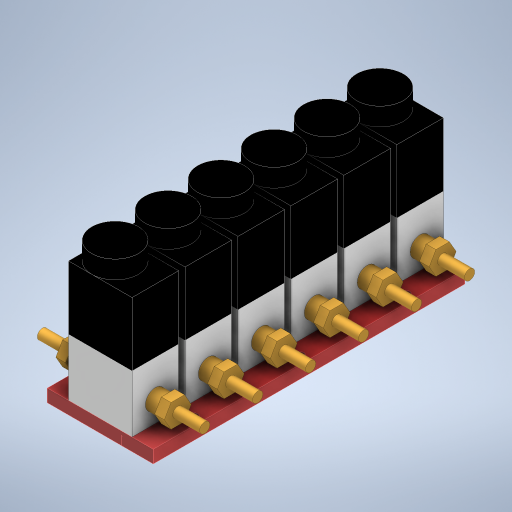
# Autodesk Inventor part: Montaje Valvulas
Saved by Autodesk Inventor 2024.2 (Build 282272000, 272)
## iProperties
Created: 2024-05-06
Part Number: Montaje Valvulas
Material: Generic
Document SubType Name: Modeling
Designer: jp.reyesf
Density: 1 g/cm^3
Appearance: Default
Author: jp.reyesf
Autodesk Inventor part; units mm, degrees
ref_plane "YZ Plane" through (0, 0, 0) normal (1, 0, 0) x (0, 1, 0)
sketch "Sketch1" plane through (0, 0, 0) normal (0, 1, 0) x (-1, 0, 0)
  line L0 (-15, 11) -> (15, 11)
  line L1 (15, 11) -> (15, -11)
  line L2 (15, -11) -> (-15, -11)
  line L3 (-15, -11) -> (-15, 11)
  line L4 (-15, 11) -> (15, -11) construction
  line L5 (15, 11) -> (-15, -11) construction
  line L6 (0, 0) -> (-10, 0)
  line L7 (-10, 7.5) -> (-10, -7.5) construction
  circle A0 centre (-10, 7.5) radius 1.7859
  circle A1 centre (-10, -7.5) radius 1.7859
  dimension "d0" = 22
  dimension "d1" = 30
  dimension "d2" = 15
  dimension "d3" = 5
  dimension "d4" = 3.5719
  constraints: 16 end point, 3 midpoint, 2 centre point, 2 coincident, 2 horizontal, 2 parallel, 1 equal radius, 1 perpendicular, 1 vertical
  measures "d0" distance of L0.end L1.end
  measures "d1" distance of L1.end L2.end
  measures "d2" distance of L7.start L7.end
  measures "d3" distance between parallel lines of L7 L3
  measures "d4" diameter of A0
extrude "Extrusion1" add sketch "Sketch1" along normal blind 27
sketch "Sketch2" plane through (0, 27, 0) normal (0, 1, 0) x (1, 0, 0)
  line L0 (15, 11) -> (-15, 11) projected
  line L1 (-15, 11) -> (-15, -11) projected
  line L2 (-15, -11) -> (15, -11) projected
  line L3 (15, -11) -> (15, 11) projected
  circle A0 centre (10, 7.5) radius 1.7859 projected
  circle A1 centre (10, -7.5) radius 1.7859 projected
  point P0 (0, 0)
extrude "Extrusion2" add sketch "Sketch2" along normal blind 30 separate body contours L3 L2 L1 L0 | A0 | A1
sketch "Sketch3" plane through (0, 57, 0) normal (0, 1, 0) x (1, 0, 0)
  circle A0 centre (-4, 0) radius 11
  line L0 (15, 11) -> (-15, 11) projected
  line L1 (-15, 11) -> (-15, -11) projected
  line L2 (-15, -11) -> (15, -11) projected
  point P0 (0, 0)
  constraints: 3 tangent, 1 centre point
extrude "Extrusion3" add sketch "Sketch3" along normal blind 8.5 contours A0 bodies 2
sketch "Sketch4" plane through (15, 0, 11) normal (1, 0, 0) x (0, 0, -1)
  line L0 (11, 0) -> (11, 10) construction
  circle A0 centre (11, 10) radius 4.7
  dimension "d11" = 10
  dimension "d12" = 9.4
  constraints: 2 end point, 1 centre point, 1 coincident, 1 vertical
  measures "d11" distance of L0.start L0.end
  measures "d12" diameter of A0
extrude "Extrusion4" cut sketch "Sketch4" against normal blind 11.4 bodies 1
ref_plane "Work Plane1" through (0, 0, 11) normal (1, 0, 0) x (0, 0, -1)
mirror "Mirror1" about plane through (0, 0, 11) normal (1, 0, 0) of "Extrusion4" bodies 1
sketch "Sketch5" plane through (-15, 0, -11) normal (-1, 0, 0) x (0, 0, 1)
  circle A0 centre (11, 10) radius 4.7 projected
  point P0 (11, 0)
extrude "Extrusion5" add sketch "Sketch5" against normal up to surface (11.4 mm away) separate body
sketch "Sketch6" plane through (-15, 10, 0) normal (-1, 0, 0) x (0, 0, 1)
  circle A0 centre (0, 0) radius 4.7 projected
  point P0 (0, -10)
extrude "Extrusion6" add sketch "Sketch6" along normal blind 10.6 bodies 3
sketch "Sketch7" plane through (-25.6, 10, 0) normal (-1, 0, 0) x (0, 0, 1)
  circle A0 centre (0, 0) radius 4.7 projected
  line L0 (3.1754, 5.5) -> (6.3509, 0)
  line L1 (6.3509, 0) -> (3.1754, -5.5)
  line L2 (3.1754, -5.5) -> (-3.1754, -5.5)
  line L3 (-3.1754, -5.5) -> (-6.3509, 0)
  line L4 (-6.3509, 0) -> (-3.1754, 5.5)
  line L5 (-3.1754, 5.5) -> (3.1754, 5.5)
  circle A1 centre (0, 0) radius 2.4
  point P0 (0, -10)
  dimension "d19" = 11
  dimension "d22" = 4.8
  constraints: 12 end point, 2 coincident, 1 centre point, 1 horizontal, 13 other
  measures "d19" distance between parallel lines of L5 L2
  measures "d22" diameter of A1
extrude "Extrusion7" add sketch "Sketch7" against normal blind 4.6 contours A0 | L0 L1 L2 L3 L4 L5 | A1 bodies 3
extrude "Extrusion8" add sketch "Sketch7" along normal blind 12.7 contours A1 bodies 3
mirror "Mirror2" about plane through (0, 0, 11) normal (1, 0, 0) bodies 3
pattern_linear "Rectangular Pattern1" count 6 spacing 25 along (0, 0, -1) bodies 2 1 3
sketch "Sketch9" plane through (0, 0, 0) normal (0, -1, 0) x (1, 0, 0)
  line L0 (15, -11) -> (-15, -11) construction
  line L1 (15, 11) -> (15, -11) construction
  line L2 (-15, 11) -> (15, 11) construction
  line L3 (-15, -11) -> (-15, 11) construction
  circle A0 centre (10, -7.5) radius 1.7859 construction
  circle A1 centre (10, 7.5) radius 1.7859 construction
  line L4 (15, -36) -> (-15, -36) construction
  line L5 (15, -14) -> (15, -36) construction
  line L6 (-15, -14) -> (15, -14) construction
  line L7 (-15, -36) -> (-15, -14) construction
  circle A2 centre (10, -32.5) radius 1.7859 construction
  circle A3 centre (10, -17.5) radius 1.7859 construction
  line L8 (15, -61) -> (-15, -61) construction
  line L9 (15, -39) -> (15, -61) construction
  line L10 (-15, -39) -> (15, -39) construction
  line L11 (-15, -61) -> (-15, -39) construction
  circle A4 centre (10, -57.5) radius 1.7859 construction
  circle A5 centre (10, -42.5) radius 1.7859 construction
  line L12 (15, -86) -> (-15, -86) construction
  line L13 (15, -64) -> (15, -86) construction
  line L14 (-15, -64) -> (15, -64) construction
  line L15 (-15, -86) -> (-15, -64) construction
  circle A6 centre (10, -82.5) radius 1.7859 construction
  circle A7 centre (10, -67.5) radius 1.7859 construction
  line L16 (15, -111) -> (-15, -111) construction
  line L17 (15, -89) -> (15, -111) construction
  line L18 (-15, -89) -> (15, -89) construction
  line L19 (-15, -111) -> (-15, -89) construction
  circle A8 centre (10, -107.5) radius 1.7859 construction
  circle A9 centre (10, -92.5) radius 1.7859 construction
  line L20 (15, -136) -> (-15, -136) construction
  line L21 (15, -114) -> (15, -136) construction
  line L22 (-15, -114) -> (15, -114) construction
  line L23 (-15, -136) -> (-15, -114) construction
  circle A10 centre (10, -132.5) radius 1.7859 construction
  circle A11 centre (10, -117.5) radius 1.7859 construction
  circle A12 centre (10, 7.5) radius 1.8859
  circle A13 centre (10, -7.5) radius 1.8859
  circle A14 centre (10, -17.5) radius 1.8859
  circle A15 centre (10, -32.5) radius 1.8859
  circle A16 centre (10, -42.5) radius 1.8859
  circle A17 centre (10, -57.5) radius 1.8859
  circle A18 centre (10, -67.5) radius 1.8859
  circle A19 centre (10, -82.5) radius 1.8859
  circle A20 centre (10, -92.5) radius 1.8859
  circle A21 centre (10, -107.5) radius 1.8859
  circle A22 centre (10, -117.5) radius 1.8859
  circle A23 centre (10, -132.5) radius 1.8859
  line L24 (-25, 11) -> (25, 11)
  line L25 (25, 11) -> (25, -136)
  line L26 (25, -136) -> (-25, -136)
  line L27 (-25, -136) -> (-25, 11)
  circle A24 centre (21, -12.5) radius 1.65
  line L28 (21, -12.5) -> (21, 11) construction
  line L29 (21, -12.5) -> (25, -12.5) construction
  line L30 (-25, -112.5) -> (-21, -112.5) construction
  line L31 (-21, -112.5) -> (-21, -136) construction
  line L32 (21, -12.5) -> (-21, -12.5) construction
  line L33 (-21, -12.5) -> (-21, -112.5) construction
  line L34 (-21, -112.5) -> (21, -112.5) construction
  line L35 (21, -112.5) -> (21, -12.5) construction
  circle A25 centre (-21, -12.5) radius 1.65
  circle A26 centre (-21, -112.5) radius 1.65
  circle A27 centre (21, -112.5) radius 1.65
  circle A28 centre (21, -62.5) radius 1.65
  circle A29 centre (-21, -62.5) radius 1.65
  line L36 (15, -11) -> (15, -12.5) construction
  line L37 (15, -12.5) -> (15, -14) construction
  dimension "d35" = 0.1
  dimension "d36" = 0
  dimension "d37" = 0
  dimension "d38" = 10
  dimension "d39" = 10
  dimension "d40" = 3.3
  dimension "d42" = 4
  constraints: 28 end point, 18 centre point, 16 equal radius, 8 equal length, 6 perpendicular, 5 point on line, 3 coincident, 3 horizontal, 2 midpoint
  measures "d35" radial gap between concentric circles of A12 A1
  measures "d36" distance between parallel lines of L24 L2
  measures "d37" distance between parallel lines of L26 L20
  measures "d38" distance between parallel lines of L25 L17
  measures "d39" distance between parallel lines of L27 L19
  measures "d40" diameter of A24
  measures "d42" distance of L28.start L29.end
extrude "Extrusion9" add sketch "Sketch9" along normal blind 6 separate body
sketch "Sketch10" plane through (0, -6, 0) normal (0, -1, 0) x (1, 0, 0)
  line L0 (-25, -136) -> (25, -136) projected
  line L1 (25, -136) -> (25, 11) projected
  line L2 (25, 11) -> (-25, 11) projected
  line L3 (-25, 11) -> (-25, -136) projected
  circle A0 centre (-21, -62.5) radius 1.65 projected
  circle A1 centre (21, -112.5) radius 1.65 projected
  circle A2 centre (-21, -12.5) radius 1.65 projected
  circle A3 centre (10, -132.5) radius 1.8859 projected
  circle A4 centre (10, -107.5) radius 1.8859 projected
  circle A5 centre (10, -82.5) radius 1.8859 projected
  circle A6 centre (10, -67.5) radius 1.8859 projected
  circle A7 centre (10, -57.5) radius 1.8859 projected
  circle A8 centre (10, -42.5) radius 1.8859 projected
  circle A9 centre (10, -32.5) radius 1.8859 projected
  circle A10 centre (10, -17.5) radius 1.8859 projected
  circle A11 centre (10, -7.5) radius 1.8859 projected
  circle A12 centre (10, 7.5) radius 1.8859 projected
  circle A13 centre (10, -92.5) radius 1.8859 projected
  circle A14 centre (10, -117.5) radius 1.8859 projected
  circle A15 centre (21, -12.5) radius 1.65 projected
  circle A16 centre (-21, -112.5) radius 1.65 projected
  circle A17 centre (21, -62.5) radius 1.65 projected
  circle A18 centre (10, -132.5) radius 3.5
  circle A19 centre (10, -117.5) radius 3.5
  circle A20 centre (10, -107.5) radius 3.5
  circle A21 centre (10, -92.5) radius 3.5
  circle A22 centre (10, -82.5) radius 3.5
  circle A23 centre (10, -67.5) radius 3.5
  circle A24 centre (10, -57.5) radius 3.5
  circle A25 centre (10, -42.5) radius 3.5
  circle A26 centre (10, -32.5) radius 3.5
  circle A27 centre (10, -17.5) radius 3.5
  circle A28 centre (10, -7.5) radius 3.5
  circle A29 centre (10, 7.5) radius 3.5
  line L4 (-25, -136) -> (25, -136) projected
  point P0 (0, 0)
  constraints: 12 centre point, 11 equal radius, 1 tangent
extrude "Extrusion10" cut sketch "Sketch10" against normal blind 4 contours A18 | A29 | A3 | A4 | A5 | A6 | A7 | A8 | A9 | A10 | A11 | A12 | A13 | A14 | A19 | A20 | A21 | A22 | A23 | A24 | A25 | A26 | A27 | A28 bodies 4
sketch "Sketch11" plane through (0, -6, 0) normal (0, -1, 0) x (1, 0, 0)
  line L0 (-6, 1) -> (-11, 1)
  line L1 (-11, 1) -> (-11, -126)
  line L2 (-11, -126) -> (-6, -126)
  line L3 (-6, -126) -> (-6, 1)
  line L4 (10, 11) -> (-25, 11) projected
  line L5 (-25, -136) -> (10, -136) projected
  line L6 (-25, 11) -> (-25, -136) projected
  point P0 (0, 0)
  dimension "d46" = 10
  dimension "d47" = 10
  dimension "d48" = 5
  dimension "d49" = 14
  constraints: 8 end point, 2 parallel, 1 horizontal, 1 perpendicular
  measures "d46" distance between parallel lines of L4 L0
  measures "d47" distance between parallel lines of L5 L2
  measures "d48" distance between parallel lines of L3 L1
  measures "d49" distance between parallel lines of L1 L6
extrude "Extrusion11" cut sketch "Sketch11" against normal blind 3 bodies 4
chamfer "Chamfer1" distance 3 angle 45 4 edges at (-6, -6, -62.5) (-8.5, -6, 1) (-11, -6, -62.5) (-8.5, -6, -126)
ref_plane "Work Plane2" through (0, -6, 0) normal (0, -1, 0) x (1, 0, 0)
body "Solid6"
body "Solid8"
body "Solid11"
body "Solid14"
body "Solid17"
body "Solid20"
body "Solid7"
body "Solid10"
body "Solid13"
body "Solid16"
body "Solid19"
body "Solid9"
body "Solid12"
body "Solid15"
body "Solid18"
body "Solid21"
body "Solid24"
body "Solid23"
body "Solid22"
body "Solid26"
body "Solid31"
body "Solid36"
body "Solid27"
body "Solid32"
body "Solid37"
body "Solid28"
body "Solid33"
body "Solid38"
body "Solid29"
body "Solid39"
body "Solid34"
body "Solid30"
body "Solid35"
body "Solid40"
body "Solid25"
